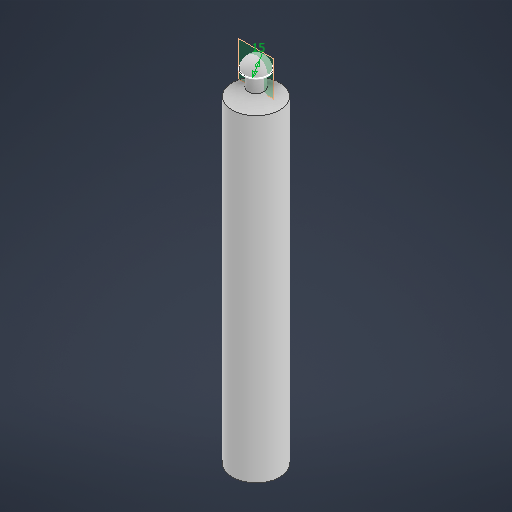
# Autodesk Inventor part: Shafts
Saved by Autodesk Inventor 2026.2 (Build 302298000, 298)
## iProperties
Created: 2025-12-10
Part Number: Shafts
Material: Generic
Document SubType Name: Modeling
Designer: Thoma
Density: 1 g/cm^3
Appearance: Default
Author: Thoma
Autodesk Inventor part; units mm, degrees
ref_plane "YZ Plane" through (0, 0, 0) normal (1, 0, 0) x (0, 1, 0)
ref_plane "XZ Plane" through (0, 0, 0) normal (0, 1, 0) x (-1, 0, 0)
ref_plane "XY Plane" through (0, 0, 0) normal (0, 0, 1) x (1, 0, 0)
sketch "Sketch4" plane through (0, 0, 0) normal (0, 0, 1) x (1, 0, 0)
  line L0 (0, 0) -> (15, 0)
  line L1 (15, 0) -> (0, 7.5)
  line L2 (0, 7.5) -> (0, 0)
  line L3 (0, 5) -> (5, 5)
  dimension "d4" = 15
  dimension "d5" = 7.5
  dimension "d6" = 2.5
  constraints: 8 end point, 2 perpendicular, 2 point on line, 1 horizontal
  measures "d4" distance of L0.start L0.end
  measures "d5" distance of L1.end L0.start
  measures "d6" distance of L1.end L3.start
revolve "Revolution1" add sketch "Sketch4" angle 360 about axis through (0, 7.5, 0) along (0, -1, 0) contours L2 L3 L1 L0
sketch "Sketch5" plane through (0, 0, 0) normal (0, -1, 0) x (1, 0, 0)
  circle A0 centre (0, 0) radius 15
  point P0 (0, 0)
  dimension "d17" = 30
  constraints: 1 centre point, 1 coincident
  measures "d17" diameter of A0
extrude "Extrusion2" add sketch "Sketch5" along normal blind 200
sketch "Sketch7" plane through (0, 5, 0) normal (0, 1, 0) x (1, 0, 0)
  circle A0 centre (0, 0) radius 5
  point P0 (0, 0)
  dimension "d18" = 10
  constraints: 1 centre point, 1 coincident
  measures "d18" diameter of A0
extrude "Extrusion4" add sketch "Sketch7" along normal blind 10
sketch "Sketch8" plane through (0, 15, 0) normal (0, 1, 0) x (1, 0, 0)
  circle A0 centre (0, 0) radius 7.5
  line L0 (0, -7.5) -> (0, 7.5)
  point P0 (0, 0)
  dimension "d19" = 15
  constraints: 2 end point, 2 point on circle, 1 centre point, 1 coincident, 1 vertical
  measures "d19" diameter of A0
ref_plane "Work Plane1" through (0, 15, 0) normal (0, 0, -1) x (-1, 0, 0)
sketch "Sketch9" plane through (0, 15, 0) normal (0, 0, -1) x (-1, 0, 0)
  line L0 (0, 0) -> (7.5, 0)
  line L1 (0, 0) -> (0, 7.5)
  circle A0 centre (0, 0) radius 7.5
  line L2 (0, 0) -> (-7.5, 0)
  point P0 (0, -15)
  dimension "d20" = 7.5
  dimension "d21" = 7.5
  constraints: 6 end point, 2 horizontal, 2 point on circle, 1 centre point, 1 coincident, 1 vertical
  measures "d20" distance of L0.start L0.end
  measures "d21" distance of L0.start L1.end
revolve "Revolution2" add sketch "Sketch9" angle 360 about axis through (0, 15, 0) along (0, 1, 0) contours L1 A0 L0
body "Solid2"
